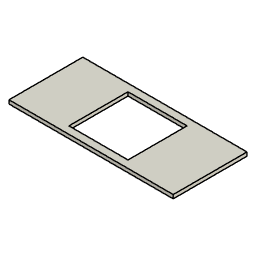
sorting_mechanism_top_panel (Autodesk Fusion 360 design; units mm, degrees)
part number: 2025-05-13-09-48-31-121
Autodesk Fusion 360 part; units mm, degrees
sketch "Sorting Mechanism Top Panel" plane through (0, 0, 0) normal (0, 0, 1) x (1, 0, 0)
  line L0 (0, 0) -> (267, 0)
  line L1 (267, 0) -> (267, 120)
  line L2 (267, 120) -> (0, 120)
  line L3 (0, 120) -> (0, 0)
  dimension "d1" = 267
  dimension "d2" = 120
  constraint horizontal L0
  constraint vertical L1
  constraint horizontal L2
  constraint vertical L3
  constraint coincident L0.start L3.end
  measures "d1" distance of L0.start L0.end
  measures "d2" distance of L0.end L1.end
extrude "Extrude1" add sketch "Sorting Mechanism Top Panel" along normal blind 6
sketch "Smartie Hopper Hole" plane through (0, 0, 6) normal (0, 0, 1) x (-1, 0, 0)
  line L0 (0, -120) -> (0, 0)
  line L1 (0, 0) -> (-267, 0)
  line L2 (-267, 0) -> (-267, -120)
  line L3 (-267, -120) -> (0, -120)
  line L4 (-85.5, -108) -> (-181.5, -108)
  line L5 (-181.5, -108) -> (-181.5, -12)
  line L6 (-181.5, -12) -> (-85.5, -12)
  line L7 (-85.5, -12) -> (-85.5, -108)
  dimension "d7" = 96
  dimension "d9" = 96
  dimension "d10" = 85.5
  dimension "d11" = 85.5
  dimension "d12" = 12
  dimension "d13" = 12
  constraint horizontal L4
  constraint vertical L5
  constraint horizontal L6
  constraint vertical L7
  measures "d7" distance of L4.start L4.end
  measures "d9" distance of L4.end L5.end
  measures "d10" distance of L0 L7
  measures "d11" distance of L2 L5
  measures "d12" distance of L3 L4
  measures "d13" distance of L1 L6
extrude "Extrude2" cut sketch "Smartie Hopper Hole" against normal blind 6 contours L4 L5 L6 L7
equation "d3 = MDF_thickness"
equation "acrylic_thickness = 3 mm" comment "Thickness of the clear acrylic panels"
equation "MDF_thickness = 6 mm" comment "Thickness of the MDF panels"
equation "d7 = smarties_feed_hole_size + 2 * acrylic_thickness"
equation "smarties_feed_hole_size = 90 mm" comment "Width of the Smarties feed hole in the Smartie Feed component"
equation "d9 = smarties_feed_hole_size + 2 * acrylic_thickness"
equation "d10 = ( 267 mm - ( smarties_feed_hole_size + 2 * acrylic_thickness ) ) / 2"
equation "d12 = ( 120 mm - ( smarties_feed_hole_size + 2 * acrylic_thickness ) ) / 2"
equation "d14 = -MDF_thickness"
named bodies: "Sorting Mechanism Top Panel"
